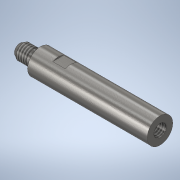
# Autodesk Inventor part: Kicker Eisen
Saved by Autodesk Inventor 2020 (Build 240168000, 168)
## iProperties
Part Number: Kicker Eisen
Material: Stahl, galvanisiert
Document SubType Name: Modeling
Designer: rYan
Mass: 21.4287 g
Surface Area: 15.1763 cm^2
Volume: 2.72978 cm^3
Density: 7.85 g/cm^3
Appearance: Galvanisiert
Author: rYan
Autodesk Inventor part; units mm, degrees
ref_plane "YZ Plane" through (0, 0, 0) normal (1, 0, 0) x (0, 1, 0)
ref_plane "XZ Plane" through (0, 0, 0) normal (0, 1, 0) x (-1, 0, 0)
ref_plane "XY Plane" through (0, 0, 0) normal (0, 0, 1) x (1, 0, 0)
sketch "Skizze1" plane through (0, 0, 0) normal (0, 0, 1) x (1, 0, 0)
  line L0 (0, 0) -> (55, 0)
  line L1 (0, 0) -> (0, 3)
  line L2 (0, 3) -> (8, 3)
  line L3 (8, 3) -> (8, 5)
  line L4 (8, 5) -> (55, 5)
  line L5 (55, 5) -> (55, 0)
  dimension "d1" = 6
  dimension "d2" = 10
  dimension "d3" = 8
  dimension "d17" = 47
  constraints: 12 end point, 2 perpendicular, 2 vertical, 1 coincident, 1 horizontal, 1 parallel
  measures "d1" diameter of L2 L0
  measures "d2" diameter of L4 L0
  measures "d3" distance of L1.end L2.end
  measures "d17" distance of L3.end L4.end
revolve "Umdrehung1" add sketch "Skizze1" angle 360 about axis through (0, 0, 0) along (1, 0, 0)
sketch "Skizze2" plane through (55, 0, 0) normal (1, 0, 0) x (0, 0, -1)
  point P0 (0, 0)
  point P1 (0, 0)
  constraints: 1 coincident
hole "Bohrung1" at (55, 0, 0) direction (-1, 0, 0) diameter 4.917 depth 13 tip angle 118 thread size "M6x1" class "6H" standard "ISO Metric profile"
sketch "Sketch3" plane through (8, 0, 0) normal (-1, 0, 0) x (0, 0, 1)
  circle A0 centre (0, 0) radius 3 projected
  circle A1 centre (0, 0) radius 2.2
  dimension "d21" = 4.4
  constraints: 1 centre point, 1 coincident
  measures "d21" diameter of A1
extrude "Extrusion1" cut sketch "Sketch3" along normal blind 1.1
chamfer "Chamfer6" distance 1.4 distance2 0.8 1 edges at (6.9, -3, 0) measured on face at (6.4, -3, 0)
chamfer "Chamfer7" distance 1.4 distance2 0.8 1 edges at (0, -3, 0) measured on face at (0.5, -3, 0)
fillet "Fillet3" radius 0.6 3 edges at (6.9, -2.2001, 0) (6.9, 0, -2.2) (8, 0, -2.2)
thread "Thread3" size "M6x1" class "6g" standard "ANSI Metric M Profile" full length
sketch "Sketch4" plane through (0, 0, 0) normal (0, 1, 0) x (-1, 0, 0)
  line L0 (-8, 5) -> (-8, -5) projected
  line L1 (-55, 5) -> (-55, -5) projected
  line L2 (-8, 5) -> (-55, 5) projected
  line L3 (-20, 5) -> (-15, 5)
  line L4 (-15, 5) -> (-15, 4.5)
  line L5 (-15, 4.5) -> (-20, 4.5)
  line L6 (-20, 4.5) -> (-20, 5)
  line L7 (-8, -5) -> (-55, -5) projected
  line L8 (-20, -5) -> (-15, -5)
  line L9 (-15, -5) -> (-15, -4.5)
  line L10 (-15, -4.5) -> (-20, -4.5)
  line L11 (-20, -4.5) -> (-20, -5)
  point P0 (0, 0)
  point P1 (-15, -5)
  point P2 (-15, 5)
  dimension "d46" = 5
  dimension "d47" = 0.5
  dimension "d48" = 5
  dimension "d49" = 0.5
  dimension "d50" = 35
  dimension "d51" = 35
  constraints: 16 end point, 4 parallel, 2 horizontal, 2 perpendicular, 2 point on line
  measures "d46" distance of L4.end L5.end
  measures "d47" distance of L3.end L4.end
  measures "d48" distance of L10.end L9.end
  measures "d49" distance of L9.end L8.end
  measures "d50" distance from line of L1 L8.start
  measures "d51" distance from line of L1 L3.start
extrude "Extrusion2" cut sketch "Sketch4" against normal through all both and the other way through all contours L4 L5 L6 L2 | L7 L11 L10 L9
